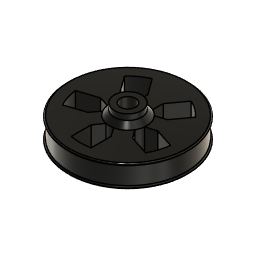
Front Wheel Without Tire v3 (Autodesk Fusion 360 design; units mm, degrees)
Autodesk Fusion 360 part; units mm, degrees
note: some values were not read from the file. Set by a fixed rule: which sketch regions a step uses.
sketch "Sketch1" plane through (0, 0, 0) normal (0, 0, 1) x (1, 0, 0)
  circle A0 centre (0, 0) radius 24
  dimension "d6" = 48
  constraint coincident A0.centre origin
  measures "d6" diameter of A0
extrude "Extrude1" add sketch "Sketch1" along normal blind 9
sketch "Sketch2" plane through (0, 0, 9) normal (0, 0, 1) x (-1, 0, 0)
  circle A0 centre (0, 0) radius 24
  circle A1 centre (0, 0) radius 3.1
  dimension "d3" = 6.2
  constraint coincident A0.centre A1.centre
  measures "d3" diameter of A1
extrude "Extrude2" cut sketch "Sketch2" against normal blind 10 contours A1
sketch "Sketch3" plane through (0, 0, 9) normal (0, 0, 1) x (-1, 0, 0)
  circle A0 centre (0, 0) radius 3.1
  circle A1 centre (0, 0) radius 24
  circle A2 centre (0, 0) radius 5.5
  dimension "d7" = 11
  constraint concentric A0 A2
  measures "d7" diameter of A2
extrude "Extrude3" add sketch "Sketch3" along normal blind 4.3 contours A2
sketch "Sketch4" plane through (0, 0, 0) normal (0, 0, -1) x (1, 0, 0)
  circle A0 centre (0, 0) radius 3.1
  circle A1 centre (0, 0) radius 24
  circle A2 centre (0, 0) radius 5.5
  dimension "d10" = 11
  constraint coincident A0.centre A1.centre
  measures "d10" diameter of A2
extrude "Extrude4" add sketch "Sketch4" along normal blind 4.3 contours A2
chamfer "Chamfer1" distance 2 angle 45 1 edges at (-5.1278, -1.9889, 0)
chamfer "Chamfer2" distance 2 angle 45 1 edges at (5.1278, -1.9889, 9)
sketch "Sketch5" plane through (0, 0, 0) normal (0, 1, 0) x (1, 0, 0)
  line L0 (-5.5, -13.3) -> (5.5, -13.3)
  line L1 (5.5, 4.3) -> (-5.5, 4.3)
  line L2 (5.5, -11) -> (7.5, -9)
  line L3 (-5.5, -11) -> (-7.5, -9)
  line L4 (-5.5, -11) -> (-5.5, -13.3)
  line L5 (5.5, -11) -> (5.5, -13.3)
  line L6 (-5.5, 2) -> (-7.5, 0)
  line L7 (5.5, 2) -> (7.5, 0)
  line L8 (5.5, 2) -> (5.5, 4.3)
  line L9 (-5.5, 2) -> (-5.5, 4.3)
  line L10 (-24, 0) -> (-24, -9)
  line L11 (24, 0) -> (24, -9)
  line L12 (1, -8.5) -> (-1, -4.25)
  line L13 (-1, -4.25) -> (1, -0.5)
  line L14 (2.5, -8.5) -> (0.5, -4.25)
  line L15 (0.5, -4.25) -> (2.5, -0.5)
  line L16 (1, -8.5) -> (2.5, -8.5)
  line L17 (1, 0) -> (3.0862, 0)
  line L18 (-24, -9) -> (-7.5, -9)
  line L19 (7.5, -9) -> (24, -9)
  line L20 (-24, 0) -> (-7.5, 0)
  line L21 (7.5, 0) -> (24, 0)
  line L22 (1, -0.5) -> (2.5, -0.5)
  dimension "d17" = 2
  dimension "d18" = 4.25
  dimension "d19" = 4.25
  dimension "d20" = 1
  dimension "d21" = 1.5
  dimension "d28" = 0.5
  dimension "d29" = 2
  constraint horizontal origin L17.start
  constraint vertical L12.start L17.start
  constraint parallel L12 L14
  constraint horizontal L12.start L14.start
  constraint horizontal L17.start L17.end
  constraint horizontal L12.end L14.end
  constraint parallel L13 L15
  constraint horizontal L22
  measures "d17" horizontal distance of L12.start L12.end
  measures "d18" vertical distance of L12.start L12.end
  measures "d19" vertical distance of L12.end L17.start
  measures "d20" distance of origin L17.start
  measures "d21" distance of L12.start L14.start
  measures "d28" distance of L17 L22
  measures "d29" horizontal distance of L12.end L13.end
sketch "Sketch7" plane through (0, 0, 0) normal (0, 0, -1) x (1, 0, 0)
  circle A0 centre (0, 0) radius 23.5
  circle A1 centre (0, 0) radius 24
  circle A2 centre (0, 0) radius 7.5
  constraint concentric A0 A1
extrude "Extrude8" cut sketch "Sketch7" against normal blind 7 from surface at -1 contours A1
chamfer "Chamfer3" distance 0.5 angle 45 2 edges at (-22.3759, -8.6788, 8) (-22.3759, 8.6788, 1)
fillet "Fillet4" radius 0.5 2 edges at (-22.3759, -8.6788, 9) (-22.3759, -8.6788, 0)
sketch "Sketch6" plane through (0, 0, 0) normal (0, 0, -1) x (1, 0, 0)
  circle A0 centre (0, 0) radius 7.5
  circle A1 centre (0, 0) radius 23.5
  arc A2 (4, 18.8185) -> (-4, 18.8185) centre (0, 0) ccw
  line L0 (0, 0) -> (4, 18.8185) construction
  line L1 (0, 0) -> (-4, 18.8185) construction
  arc A3 (1.5593, 7.3361) -> (-1.5593, 7.3361) centre (0, 0) ccw
  line L2 (-4, 18.8185) -> (-4, 10.8185)
  line L3 (-4, 10.8185) -> (-1.5593, 7.3361)
  line L4 (4, 18.8185) -> (4, 10.8185)
  line L5 (4, 10.8185) -> (1.5593, 7.3361)
  dimension "d38" = 24
  dimension "d39" = 4
  dimension "d40" = 4
  dimension "d45" = 8
  dimension "d46" = 8
  constraint coincident A0.centre A1.centre
  constraint coincident L0 A3.start
  constraint coincident L1 A3.end
  constraint coincident A0 A3.end
  constraint vertical L2
  constraint vertical L4
  measures "d38" angle of L0 L1
  measures "d39" horizontal distance of A2.end A0.centre
  measures "d40" horizontal distance of A0.centre A2.start
  measures "d45" distance of A2.start L4.end
  measures "d46" distance of A2.end L2.end
extrude "Extrude7" cut sketch "Sketch6" against normal blind 10 contours A0 A2 A3 L2 L3 L4 L5
pattern_circular "C-Pattern2" count 5 over 360 about axis through (0, 0, 1.75) along (0, 0, 1) of "Extrude7"
